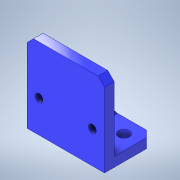
# Autodesk Inventor part: Vertical TOF mount
Saved by Autodesk Inventor 2022.6 (Build 266554000, 554)
## iProperties
Created: 2024-10-19
Part Number: Vertical TOF mount
Material: Generic
Document SubType Name: Modeling
Designer: Asus
Density: 1 g/cm^3
Appearance: Blue - Wall Paint - Glossy
Author: Asus
Autodesk Inventor part; units mm, degrees
ref_plane "XY Plane" through (0, 0, 0) normal (0, 0, 1) x (1, 0, 0)
sketch "Sketch1" plane through (0, 0, 0) normal (0, 0, 1) x (1, 0, 0)
  line L0 (0, 0) -> (24, 0)
  line L1 (24, 0) -> (24, 20)
  line L2 (24, 20) -> (0, 20)
  line L3 (0, 20) -> (0, 0)
  line L4 (0, 20) -> (24, 20)
  line L5 (24, 20) -> (24, 20)
  line L6 (24, 20) -> (0, 20)
  line L7 (0, 20) -> (0, 20)
  dimension "d0" = 24
  dimension "d1" = 20
  dimension "d47" = 0
  dimension "d48" = 24
  constraints: 16 end point, 4 equal length, 2 horizontal, 2 perpendicular
  measures "d0" distance of L2.end L1.end
  measures "d1" distance of L1.end L0.end
  measures "d47" distance between parallel lines of L2 L6
  measures "d48" distance of L5.end L6.end
extrude "Extrusion1" add sketch "Sketch1" along normal blind 3
ref_plane "Work Plane1" through (12, 0, 0) normal (1, 0, 0) x (0, 1, 0)
ref_plane "Work Plane2" through (0, 23, 0) normal (0, 1, 0) x (-1, 0, 0)
sketch "Sketch5" plane through (0, 20, 0) normal (0, 1, 0) x (1, 0, 0)
  line L0 (0, 0) -> (0, -3) projected
  line L1 (24, 0) -> (24, -3) projected
  line L2 (0, 0) -> (24, 0)
  line L3 (24, 0) -> (24, -3)
  line L4 (24, -3) -> (0, -3)
  line L5 (0, -3) -> (0, 0)
  constraints: 8 end point, 2 parallel, 1 horizontal, 1 perpendicular
extrude "Extrusion4" add sketch "Sketch5" along normal blind 5
sketch "Sketch6" plane through (0, 0, 3) normal (0, 0, 1) x (1, 0, 0)
  line L0 (0, 0) -> (0, 25) projected
  line L1 (24, 0) -> (24, 25) projected
  line L2 (0, 25) -> (24, 25)
  line L3 (24, 25) -> (24, 22)
  line L4 (24, 22) -> (0, 22)
  line L5 (0, 22) -> (0, 25)
  point P0 (24, 25)
  point P1 (0, 22)
  dimension "d51" = 3
  constraints: 8 end point, 2 parallel, 1 horizontal, 1 perpendicular, 1 point on line
  measures "d51" distance of L2.end L3.end
extrude "Extrusion5" add sketch "Sketch6" against normal blind 15
sketch "Sketch7" plane through (0, 25, 0) normal (0, 1, 0) x (1, 0, 0)
  line L0 (0, -3) -> (0, 12) projected
  line L1 (0, 12) -> (24, 12) projected
  line L2 (4.5, 7.5) -> (19.5, 7.5) construction
  line L3 (0, 0) -> (24, 0) projected
  point P0 (12, 7.5)
  dimension "d54" = 15
  dimension "d55" = 4.5
  dimension "d56" = 4.5
  constraints: 2 end point, 1 horizontal, 1 midpoint
  measures "d54" distance of L2.end L2.start
  measures "d55" distance from line of L2.start L0
  measures "d56" distance from line of L1 L2.start
hole "Hole3" at (4.5, 25, -7.5) at (19.5, 25, -7.5) direction (0, -1, 0) diameter 3.4 end through all
chamfer "Chamfer1" distance 2 angle 45 4 edges at (0, 23.5, -12) (24, 23.5, -12) (24, 0, 1.5) (0, 0, 1.5)
sketch "Sketch10" plane through (12, 0, 0) normal (1, 0, 0) x (0, 1, 0)
  line L0 (2, 3) -> (25, 3) projected
  line L1 (25, 3) -> (25, -10) projected
  line L2 (22, 0) -> (22, -10) projected
  line L3 (2, 0) -> (22, 0) projected
  line L4 (22, -12) -> (7, 0)
  line L5 (2, 3) -> (2, 0) projected
  line L6 (22, -10) -> (25, -10) projected
  dimension "d87" = 15
  constraints: 2 end point, 1 point on line
  measures "d87" distance from line of L2 L4.end
extrude "Rib1" add sketch "Sketch10" along normal mid plane 2 rib yes fills toward (14.5312, -5.961) open curves L4
sketch "Sketch11" plane through (0, 0, 3) normal (0, 0, 1) x (1, 0, 0)
  line L0 (0, 25) -> (24, 25) projected
  line L1 (0, 2) -> (0, 25) projected
  line L2 (2, 0) -> (0, 2) projected
  line L3 (2, 0) -> (22, 0) projected
  line L4 (24, 2) -> (22, 0) projected
  line L5 (24, 2) -> (24, 25) projected
  circle A0 centre (20.25, 15) radius 1.2
  circle A1 centre (3.75, 15) radius 1.2
  line L6 (2, 0) -> (22, 0) construction
  line L7 (12, 0) -> (12, 25) construction
  circle A2 centre (20.25, 15) radius 2
  circle A3 centre (3.75, 15) radius 2
  line L8 (14.5, 0) -> (9.5, 0)
  line L9 (9.5, 0) -> (9.5, 2)
  line L10 (9.5, 2) -> (14.5, 2)
  line L11 (14.5, 2) -> (14.5, 0)
  line L12 (12, 0) -> (12, 3.7497) construction
  point P0 (0, 0)
  dimension "d88" = 2.4
  dimension "d89" = 15
  dimension "d91" = 16.5
  dimension "d92" = 4
  dimension "d95" = 5
  dimension "d96" = 2
  constraints: 12 end point, 4 centre point, 3 midpoint, 2 parallel, 2 symmetric about line, 1 coincident, 1 collinear, 1 equal radius, 1 horizontal, 1 horizontal alignment, 1 perpendicular, 1 point on line, 1 vertical, 1 other
  measures "d88" diameter of A0
  measures "d89" distance from line of L3 A0.centre
  measures "d91" distance of A1.centre A0.centre
  measures "d92" diameter of A2
  measures "d95" distance of L9.end L10.end
  measures "d96" distance of L8.end L9.end
extrude "Extrusion7" [suppressed]
hole "Hole4" at (20.25, 15, 3) at (3.75, 15, 3) direction (0, 0, -1) diameter 2.4 end through all
body "Solid1"
